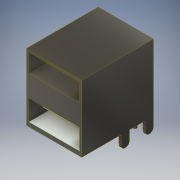
# Autodesk Inventor part: USBA_CNC
Saved by Autodesk Inventor 2016 (Build 200138000, 138)
## iProperties
Created: 2017-03-02
Part Number: USBA_CNC
Material: Generic
Document SubType Name: Modeling
Designer: jfixelle
Density: 1 g/cm^3
Appearance: Silver
Author: jfixelle
Autodesk Inventor part; units mm, degrees
ref_plane "YZ Plane" through (0, 0, 0) normal (1, 0, 0) x (0, 1, 0)
ref_plane "XZ Plane" through (0, 0, 0) normal (0, 1, 0) x (-1, 0, 0)
ref_plane "XY Plane" through (0, 0, 0) normal (0, 0, 1) x (1, 0, 0)
sketch "Sketch1" plane through (0, 0, 0) normal (0, 0, 1) x (1, 0, 0)
  line L0 (-6.55, 7.9) -> (6.55, 7.9)
  line L1 (6.55, 7.9) -> (6.55, -7.9)
  line L2 (6.55, -7.9) -> (-6.55, -7.9)
  line L3 (-6.55, -7.9) -> (-6.55, 7.9)
  point P0 (0, 0)
  dimension "d0" = 13.1
  dimension "d1" = 15.8
  dimension "d2" = 7.9
  dimension "d3" = 6.55
  constraints: 8 end point, 2 parallel, 1 horizontal, 1 perpendicular
  measures "d0" distance of L0.start L0.end
  measures "d1" distance of L0.end L1.end
  measures "d2" distance from line of point (0, 0) L0
  measures "d3" distance from line of point (0, 0) L1
extrude "Extrusion1" add sketch "Sketch1" along normal blind 17
sketch "Sketch2" plane through (0, 0, 17) normal (0, 0, 1) x (1, 0, 0)
  line L0 (-6, 7.4) -> (6, 7.4)
  line L1 (6, 7.4) -> (6, 3)
  line L2 (6, 3) -> (-6, 3)
  line L3 (-6, 3) -> (-6, 7.4)
  line L4 (-6, -2) -> (6, -2)
  line L5 (6, -2) -> (6, -6.9)
  line L6 (6, -6.9) -> (-6, -6.9)
  line L7 (-6, -6.9) -> (-6, -2)
  line L8 (-6.55, -7.9) -> (6.55, -7.9) projected
  line L9 (6.55, 7.9) -> (-6.55, 7.9) projected
  point P0 (0, 0)
  dimension "d6" = 12
  dimension "d7" = 12
  dimension "d8" = 6
  dimension "d9" = 1
  dimension "d10" = 0.5
  dimension "d11" = 5
  dimension "d12" = 2
  constraints: 16 end point, 4 parallel, 2 horizontal, 2 perpendicular, 1 point on line
  measures "d6" distance of L0.start L0.end
  measures "d7" distance of L4.start L4.end
  measures "d8" distance from line of point (0, 0) L5
  measures "d9" distance between parallel lines of L8 L6
  measures "d10" distance between parallel lines of L9 L0
  measures "d11" distance between parallel lines of L4 L2
  measures "d12" distance from line of point (0, 0) L4
extrude "Extrusion2" cut sketch "Sketch2" against normal blind 10
sketch "Sketch3" plane through (0, 0, 7) normal (0, 0, 1) x (1, 0, 0)
  line L0 (-4.6506, 6.4578) -> (5.055, 6.4578)
  line L1 (5.055, 6.4578) -> (5.055, 5.3457)
  line L2 (5.055, 5.3457) -> (-4.6506, 5.3457)
  line L3 (-4.6506, 5.3457) -> (-4.6506, 6.4578)
  line L4 (-4.6506, -3.0962) -> (5.055, -3.0962)
  line L5 (5.055, -3.0962) -> (5.055, -4.2083)
  line L6 (5.055, -4.2083) -> (-4.6506, -4.2083)
  line L7 (-4.6506, -4.2083) -> (-4.6506, -3.0962)
  point P0 (0, 0)
  constraints: 16 end point, 4 parallel, 2 horizontal, 2 perpendicular, 2 point on line
extrude "Extrusion3" add sketch "Sketch3" along normal blind 8
sketch "Sketch4" plane through (6.55, -7.9, 0) normal (1, 0, 0) x (0, 0, -1)
  line L0 (-7.7, 2.838) -> (-5.7, 2.838)
  line L1 (-5.7, 2.838) -> (-5.7, -3.2)
  line L2 (-5.7, -3.2) -> (-7.7, -3.2)
  line L3 (-7.7, -3.2) -> (-7.7, 2.838)
  line L4 (-17, 0) -> (-17, 15.8) projected
  line L5 (-2.02, 6.1684) -> (-0.02, 6.1684)
  line L6 (-0.02, 6.1684) -> (-0.02, -3.2)
  line L7 (-0.02, -3.2) -> (-2.02, -3.2)
  line L8 (-2.02, -3.2) -> (-2.02, 6.1684)
  arc A0 (-7.7, -2.2) -> (-5.7, -2.2) centre (-6.7, -2.2) ccw
  arc A1 (-2.02, -2.2) -> (-0.02, -2.2) centre (-1.02, -2.2) ccw
  point P0 (0, 7.9)
  dimension "d17" = 2
  dimension "d18" = 9.3
  dimension "d19" = 2
  dimension "d20" = 3.68
  dimension "d21" = 3.2
  dimension "d22" = 0
  constraints: 16 end point, 6 tangent, 4 parallel, 4 point on circle, 4 point on line, 2 centre point, 2 horizontal, 2 perpendicular
  measures "d17" distance of L1.end L2.end
  measures "d18" distance between parallel lines of L4 L3
  measures "d19" distance of L6.end L7.end
  measures "d20" distance between parallel lines of L8 L1
  measures "d21" distance from line of L2 L4.start
  measures "d22" distance between parallel lines of L7 L2
extrude "Extrusion4" add sketch "Sketch4" against normal blind 0.5 contours L0 L1 A0 L3 | L5 L6 A1 L8
sketch "Sketch5" plane through (-6.55, -7.9, 0) normal (0, -1, 0) x (1, 0, 0)
  line L0 (13.8244, 1.33) -> (1.8735, 1.33) construction
  line L1 (13.8244, 3.95) -> (1.8735, 3.95) construction
  line L2 (13.1, 7.7) -> (12.6, 7.7) projected
  circle A0 centre (5.55, 1.33) radius 0.4
  circle A1 centre (5.55, 3.95) radius 0.4
  circle A2 centre (7.55, 1.33) radius 0.4
  circle A3 centre (7.55, 3.95) radius 0.4
  circle A4 centre (3.05, 1.33) radius 0.4
  circle A5 centre (3.05, 3.95) radius 0.4
  circle A6 centre (10.05, 3.95) radius 0.4
  circle A7 centre (10.05, 1.33) radius 0.4
  point P0 (6.55, 0)
  dimension "d25" = 2.62
  dimension "d26" = 3.75
  dimension "d27" = 2
  dimension "d28" = 1
  dimension "d29" = 2
  dimension "d30" = 1
  dimension "d31" = 2.5
  dimension "d32" = 2.5
  dimension "d33" = 2.5
  dimension "d34" = 2.5
  dimension "d35" = 0.8
  dimension "d36" = 0.8
  dimension "d37" = 0.8
  dimension "d38" = 0.8
  dimension "d39" = 0.8
  dimension "d40" = 0.8
  dimension "d41" = 0.8
  dimension "d42" = 0.8
  constraints: 8 centre point, 8 point on line, 4 end point, 2 horizontal
  measures "d25" distance between parallel lines of L1 L0
  measures "d26" distance between parallel lines of L2 L1
  measures "d27" distance of A0.centre A2.centre
  measures "d28" horizontal distance of point (6.55, 0) A0.centre
  measures "d29" distance of A3.centre A1.centre
  measures "d30" horizontal distance of point (6.55, 0) A1.centre
  measures "d31" distance of A6.centre A3.centre
  measures "d32" distance of A2.centre A7.centre
  measures "d33" distance of A0.centre A4.centre
  measures "d34" distance of A1.centre A5.centre
  measures "d35" diameter of A1
  measures "d36" diameter of A5
  measures "d37" diameter of A4
  measures "d38" diameter of A0
  measures "d39" diameter of A2
  measures "d40" diameter of A3
  measures "d41" diameter of A7
  measures "d42" diameter of A6
extrude "Extrusion5" add sketch "Sketch5" along normal blind 3.2
mirror "Mirror1" about plane through (0, 0, 0) normal (1, 0, 0) of "Extrusion4"
body "Solid1"
